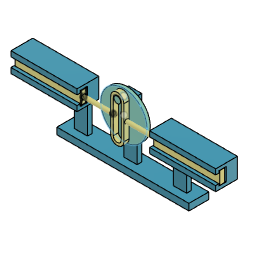
Scotch Yoke Mechanism v9 (Autodesk Fusion 360 design; units mm, degrees)
Autodesk Fusion 360 part; units mm, degrees
sketch "holder base" plane through (0, 0, 0) normal (0, 0, 1) x (1, 0, 0) in component "Holder"
  line L0 (-100, -15) -> (100, -15)
  line L1 (100, -15) -> (100, 15)
  line L2 (100, 15) -> (-100, 15)
  line L3 (-100, 15) -> (-100, -15)
  line L4 (-100, -15) -> (100, 15) construction
  line L5 (100, -15) -> (-100, 15) construction
  constraint horizontal L0
  constraint perpendicular L0 L1
  constraint parallel L0 L2
  constraint parallel L1 L3
  constraint coincident L4 origin
  constraint coincident L5 origin
extrude "Extrude1" add sketch "holder base" along normal blind 10 makes body 1 in component "Holder"
sketch "crank holder base" plane through (0, 0, 10) normal (0, 0, 1) x (-1, 0, 0) in component "Holder"
  line L0 (100, -15) -> (100, 15)
  line L1 (100, 15) -> (-100, 15)
  line L2 (-100, 15) -> (-100, -15)
  line L3 (-100, -15) -> (100, -15)
  line L4 (-10, 3.5) -> (10, 3.5)
  line L5 (10, 3.5) -> (10, -3.5)
  line L6 (10, -3.5) -> (-10, -3.5)
  line L7 (-10, -3.5) -> (-10, 3.5)
  line L8 (-10, 3.5) -> (10, -3.5) construction
  line L9 (10, 3.5) -> (-10, -3.5) construction
  dimension "d3" = 20
  dimension "d4" = 7
  constraint horizontal L4
  constraint perpendicular L4 L5
  constraint parallel L4 L6
  constraint parallel L5 L7
  constraint coincident L8 origin
  constraint coincident L9 origin
  measures "d3" distance of L5.end L6.end
  measures "d4" distance of L4.end L5.end
extrude "Extrude2" add sketch "crank holder base" along normal blind 150 contours L4 L5 L6 L7 bodies 1 in component "Holder"
sketch "slider holder base" plane through (0, 0, 10) normal (0, 0, 1) x (-1, 0, 0) in component "Holder"
  line L0 (-10, -3.5) -> (-10, 3.5)
  line L1 (-10, 3.5) -> (10, 3.5)
  line L2 (10, 3.5) -> (10, -3.5)
  line L3 (10, -3.5) -> (-10, -3.5)
  line L4 (100, -15) -> (100, 15)
  line L5 (100, 15) -> (-100, 15)
  line L6 (-100, 15) -> (-100, -15)
  line L7 (-100, -15) -> (100, -15)
  line L8 (-85, 3.5) -> (-65, 3.5)
  line L9 (-65, 3.5) -> (-65, -3.5)
  line L10 (-65, -3.5) -> (-85, -3.5)
  line L11 (-85, -3.5) -> (-85, 3.5)
  line L12 (-85, 3.5) -> (-65, -3.5) construction
  line L13 (-65, 3.5) -> (-85, -3.5) construction
  line L14 (0, -15) -> (0, 15)
  line L15 (65, -3.5) -> (85, -3.5)
  line L16 (85, 3.5) -> (65, 3.5)
  line L17 (85, -3.5) -> (85, 3.5)
  line L18 (65, 3.5) -> (65, -3.5)
  point P0 (-75, 0)
  dimension "d7" = 20
  dimension "d8" = 7
  constraint horizontal L8
  constraint perpendicular L8 L9
  constraint parallel L8 L10
  constraint parallel L9 L11
  constraint coincident L12 P0
  constraint coincident L13 P0
  constraint midpoint L7 L14.start
  constraint midpoint L5 L14.end
  constraint symmetric L8.start L14 L16.start
  constraint symmetric L8.end L14 L16.end
  constraint symmetric L9.end L14 L15.start
  constraint symmetric L10.end L14 L15.end
  measures "d7" distance of L9.end L10.end
  measures "d8" distance of L8.end L9.end
extrude "Extrude3" add sketch "slider holder base" along normal blind 110 contours L8 L9 L10 L11 | L15 L16 L17 L18 bodies 1 in component "Holder"
sketch "crank holder" plane through (0, -3.5, 0) normal (0, -1, 0) x (1, 0, 0) in component "Holder"
  line L0 (-10, 10) -> (10, 10)
  line L1 (10, 10) -> (10, 160)
  line L2 (10, 160) -> (-10, 160)
  line L3 (-10, 160) -> (-10, 10)
  circle A0 centre (0, 135) radius 5
  dimension "d11" = 10
  measures "d11" diameter of A0
extrude "Extrude4" add sketch "crank holder" along normal blind 10 contours A0 bodies 1 in component "Holder"
sketch "crank" plane through (0, -13.5, 0) normal (0, -1, 0) x (1, 0, 0) in component "Crank"
  circle A0 centre (0, 135) radius 5
  circle A1 centre (0, 135) radius 35
  circle A2 centre (0, 160) radius 5
  dimension "d14" = 10
  constraint concentric A0 A1
  measures "d14" diameter of A2
extrude "Extrude1'" add sketch "crank" against normal blind 5 separate body contours A1 | A2 makes body 2 in component "Crank"
move_face "OffsetFaces1" offset -0.3 1 faces at (-4.6985, -10.1667, 133.2899) on bodies 1 in component "Holder"
extrude "Extrude2'" add sketch "crank" along normal blind 10 contours A2 bodies 2 in component "Crank"
sketch "slider holder side" plane through (0, -3.5, 0) normal (0, -1, 0) x (1, 0, 0) in component "Holder"
  line L0 (-85, 10) -> (-65, 10)
  line L1 (-65, 10) -> (-65, 120)
  line L2 (-65, 120) -> (-85, 120)
  line L3 (-85, 120) -> (-85, 10)
  line L4 (-55, 120) -> (-155, 120)
  line L5 (-155, 120) -> (-155, 150)
  line L6 (-155, 150) -> (-55, 150)
  line L7 (-55, 150) -> (-55, 120)
  line L8 (0, 160) -> (0, 10)
  line L9 (155, 150) -> (55, 150)
  line L10 (55, 150) -> (55, 120)
  line L11 (55, 120) -> (155, 120)
  line L12 (155, 120) -> (155, 150)
  line L13 (-155, 150) -> (-55, 150)
  line L14 (-55, 150) -> (-55, 145)
  line L15 (-55, 145) -> (-155, 145)
  line L16 (-155, 145) -> (-155, 150)
  line L17 (-55, 120) -> (-155, 120)
  line L18 (-155, 120) -> (-155, 125)
  line L19 (-155, 125) -> (-55, 125)
  line L20 (-55, 125) -> (-55, 120)
  line L21 (55, 145) -> (155, 145)
  line L22 (155, 125) -> (55, 125)
  dimension "d20" = 100
  dimension "d21" = 30
  dimension "d24" = 5
  dimension "d25" = 5
  constraint horizontal L4
  constraint vertical L5
  constraint horizontal L6
  constraint vertical L7
  constraint vertical L8
  constraint symmetric L4.start L8 L10.end
  constraint symmetric L4.end L8 L11.end
  constraint symmetric L5.end L8 L9.start
  constraint symmetric L6.end L8 L9.end
  constraint horizontal L13
  constraint vertical L14
  constraint horizontal L15
  constraint vertical L16
  constraint coincident L7 L14.end
  constraint horizontal L17
  constraint vertical L18
  constraint horizontal L19
  constraint vertical L20
  constraint symmetric L8 L14.end L21.start
  constraint symmetric L8 L15.end L21.end
  constraint symmetric L8 L18.end L22.start
  constraint symmetric L8 L19.end L22.end
  measures "d20" distance of L4.start L4.end
  measures "d21" distance of L4.start L6.end
  measures "d24" distance of L5.end L15.end
  measures "d25" distance of L4.start L19.end
extrude "Extrude5" add sketch "slider holder side" against normal blind 7 contours L2 L4 L5 L7 L17 L18 L19 L20 | L5 L7 L15 L19 | L5 L6 L7 L13 L14 L15 L16 | L9 L10 L12 L21 | L10 L12 L21 L22 | L10 L11 L12 L22 bodies 1 in component "Holder"
extrude "Extrude6" add sketch "slider holder side" along normal blind 20 contours L2 L4 L5 L7 L17 L18 L19 L20 | L5 L6 L7 L13 L14 L15 L16 | L9 L10 L12 L21 | L10 L11 L12 L22 bodies 1 in component "Holder"
sketch "slider center" plane through (0, -23.5, 0) normal (0, -1, 0) x (1, 0, 0) in component "Slider"
  circle A0 centre (0, 160) radius 5
  line L0 (0, 170) -> (0, 100)
  line L1 (-10, 160) -> (-10, 110)
  line L2 (0, 100) -> (0, 170) construction
  line L3 (10, 160) -> (10, 110)
  line L4 (-10, 135) -> (10, 135) construction
  arc A1 (-6, 110) -> (6, 110) centre (0, 110) ccw
  line L5 (6, 160) -> (6, 110)
  arc A2 (6, 160) -> (-6, 160) centre (0, 160) ccw
  line L6 (-6, 110) -> (-6, 160)
  arc A3 (-10, 110) -> (10, 110) centre (0, 110) ccw
  line L7 (10, 160) -> (10, 110)
  arc A4 (10, 160) -> (-10, 160) centre (0, 160) ccw
  line L8 (-10, 110) -> (-10, 160)
  dimension "d29" = 70
  constraint vertical L0
  constraint vertical L1
  constraint vertical L2
  constraint coincident L1 L4.start
  constraint coincident L3 L4.end
  constraint tangent A1 L6
  constraint tangent A1 L5
  constraint tangent L5 A2
  constraint tangent A2 L6
  constraint tangent L7 A4
  constraint tangent A3 L8
  constraint tangent A3 L7
  constraint tangent A4 L8
  measures "d29" distance of L0.start L0.end
extrude "Extrude1''" add sketch "slider center" against normal blind 8 separate body contours L0 L1 A1 A2 L6 A3 A4 L8 | L0 L3 A1 L5 A2 A3 L7 A4 makes body 3
sketch "Sketch2" plane through (10, 0, 0) normal (1, 0, 0) x (0, 1, 0) in component "Slider"
  line L0 (-23.5, 160) -> (-23.5, 110)
  line L1 (-23.5, 110) -> (-15.5, 110)
  line L2 (-15.5, 110) -> (-15.5, 160)
  line L3 (-15.5, 160) -> (-23.5, 160)
copy_body "CutPasteBodies1" bodies 3 removing the originals makes body 4 in component "Slider"
sketch "slider right link" plane through (10, 0, 0) normal (1, 0, 0) x (0, 1, 0) in component "Slider"
  line L0 (-19.5, 160) -> (-19.5, 110) construction
  circle A0 centre (-19.5, 135) radius 3
  dimension "d34" = 6
  constraint vertical L0
  constraint midpoint L0 A0.centre
  measures "d34" diameter of A0
extrude "Extrude1'''" add sketch "slider right link" along normal blind 45 bodies 4 in component "Slider"
sketch "slider left link" plane through (-10, 0, 0) normal (-1, 0, 0) x (0, -1, 0) in component "Slider"
  line L0 (23.5, 110) -> (23.5, 160)
  line L1 (23.5, 160) -> (15.5, 160)
  line L2 (15.5, 160) -> (15.5, 110)
  line L3 (15.5, 110) -> (23.5, 110)
  line L4 (19.5, 160) -> (19.5, 110) construction
  circle A0 centre (19.5, 135) radius 3
  dimension "d37" = 6
  constraint midpoint L1 L4.start
  constraint midpoint L3 L4.end
  constraint midpoint L4 A0.centre
  measures "d37" diameter of A0
extrude "Extrude2''" add sketch "slider left link" along normal blind 45 contours A0 bodies 4 in component "Slider"
sketch "slider left" plane through (-55, 0, 0) normal (-1, 0, 0) x (0, -1, 0) in component "Slider"
  circle A0 centre (19.5, 135) radius 3
  line L0 (23.5, 125) -> (15.5, 125)
  line L1 (15.5, 125) -> (15.5, 145)
  line L2 (15.5, 145) -> (23.5, 145)
  line L3 (23.5, 145) -> (23.5, 125)
  line L4 (23.5, 125) -> (15.5, 145) construction
  line L5 (15.5, 125) -> (23.5, 145) construction
  point P0 (19.5, 135)
  dimension "d40" = 8
  dimension "d41" = 20
  constraint horizontal L0
  constraint perpendicular L0 L1
  constraint parallel L0 L2
  constraint parallel L1 L3
  constraint coincident L4 P0
  constraint coincident L5 P0
  constraint coincident P0 A0.centre
  measures "d40" distance of L1.end L2.end
  measures "d41" distance of L0.end L1.end
extrude "Extrude4'" add sketch "slider left" along normal blind 100 contours A0 | L0 L1 L2 L3 bodies 4 in component "Slider"
sketch "slider right" plane through (55, 0, 0) normal (1, 0, 0) x (0, 1, 0) in component "Slider"
  circle A0 centre (-19.5, 135) radius 3
  line L0 (-15.5, 125) -> (-23.5, 125)
  line L1 (-23.5, 125) -> (-23.5, 145)
  line L2 (-23.5, 145) -> (-15.5, 145)
  line L3 (-15.5, 145) -> (-15.5, 125)
  line L4 (-15.5, 125) -> (-23.5, 145) construction
  line L5 (-23.5, 125) -> (-15.5, 145) construction
  point P0 (-19.5, 135)
  dimension "d46" = 8
  dimension "d47" = 20
  constraint horizontal L0
  constraint perpendicular L0 L1
  constraint parallel L0 L2
  constraint parallel L1 L3
  constraint coincident L4 P0
  constraint coincident L5 P0
  constraint coincident P0 A0.centre
  measures "d46" distance of L1.end L2.end
  measures "d47" distance of L0.end L1.end
extrude "Extrude5'" add sketch "slider right" along normal blind 100 contours A0 | L0 L1 L2 L3 bodies 4 in component "Slider"
move_face "OffsetFaces1'" offset -0.3 4 faces at (88.3333, -23.5, 131.6667) (88.3333, -20.8333, 145) (88.3333, -15.5, 138.3333) (88.3333, -18.1667, 125) on bodies 4 in component "Slider"
move_face "OffsetFaces2" offset -0.3 4 faces at (-88.3333, -23.5, 138.3333) (-121.6667, -20.8333, 145) (-88.3333, -20.8333, 125) (-88.3333, -15.5, 131.6667) on bodies 4 in component "Slider"
extrude "Extrude7" add 1 faces at (-121.6667, -3.5, 131.6667) along direction (0, -1, 0) blind 10 on bodies 1 bodies 1 in component "Holder"
extrude "Extrude8" add 1 faces at (121.6667, -3.5, 131.6667) along direction (0, -1, 0) blind 10 on bodies 1 bodies 1 in component "Holder"
extrude "Extrude9" add 4 faces at (-121.6667, -23.5, 148.3333) (-121.6667, -23.5, 123.3333) (88.3333, -23.5, 148.3333) (88.3333, -23.5, 123.3333) along direction (0, -1, 0) blind 6 on bodies 1 bodies 1 in component "Holder"
sketch "slider rail right bottom" plane through (0, 0, 125) normal (0, 0, 1) x (-1, 0, 0) in component "Holder"
  line L0 (-155, 13.5) -> (-55, 13.5)
  line L1 (-55, 13.5) -> (-55, 29.5)
  line L2 (-55, 29.5) -> (-155, 29.5)
  line L3 (-155, 29.5) -> (-155, 13.5)
  line L4 (-155, 29.5) -> (-55, 29.5)
  line L5 (-55, 29.5) -> (-55, 24.5)
  line L6 (-55, 24.5) -> (-155, 24.5)
  line L7 (-155, 24.5) -> (-155, 29.5)
  dimension "d58" = 100
  dimension "d59" = 5
  constraint horizontal L4
  constraint vertical L5
  constraint horizontal L6
  constraint vertical L7
  constraint coincident L2.end L3.start
  measures "d58" distance of L2.end L1.end
  measures "d59" distance of L2.end L6.end
sketch "slider rail right top" plane through (0, 0, 145) normal (0, 0, -1) x (1, 0, 0) in component "Holder"
  line L0 (55, 13.5) -> (155, 13.5)
  line L1 (155, 13.5) -> (155, 29.5)
  line L2 (155, 29.5) -> (55, 29.5)
  line L3 (55, 29.5) -> (55, 13.5)
  line L4 (155, 29.5) -> (55, 29.5)
  line L5 (55, 29.5) -> (55, 24.5)
  line L6 (55, 24.5) -> (155, 24.5)
  line L7 (155, 24.5) -> (155, 29.5)
  dimension "d60" = 100
  dimension "d61" = 5
  constraint horizontal L4
  constraint vertical L5
  constraint horizontal L6
  constraint vertical L7
  constraint coincident L1.end L2.start
  measures "d60" distance of L1.end L2.end
  measures "d61" distance of L1.end L6.end
extrude "Extrude10" add sketch "slider rail right bottom" along normal blind 3 contours L1 L2 L3 L4 L5 L6 L7 bodies 1 in component "Holder"
extrude "Extrude11" add sketch "slider rail right top" along normal blind 3 contours L1 L2 L3 L4 L5 L6 L7 bodies 1 in component "Holder"
sketch "slider rail left bottom" plane through (0, 0, 125) normal (0, 0, 1) x (-1, 0, 0) in component "Holder"
  line L0 (55, 13.5) -> (155, 13.5)
  line L1 (155, 13.5) -> (155, 29.5)
  line L2 (155, 29.5) -> (55, 29.5)
  line L3 (55, 29.5) -> (55, 13.5)
  line L4 (155, 29.5) -> (55, 29.5)
  line L5 (55, 29.5) -> (55, 24.5)
  line L6 (55, 24.5) -> (155, 24.5)
  line L7 (155, 24.5) -> (155, 29.5)
  dimension "d66" = 100
  dimension "d67" = 5
  constraint horizontal L4
  constraint vertical L5
  constraint horizontal L6
  constraint vertical L7
  constraint coincident L1.end L2.start
  measures "d66" distance of L1.end L2.end
  measures "d67" distance of L1.end L6.end
sketch "slider rail left top" plane through (0, 0, 145) normal (0, 0, -1) x (1, 0, 0) in component "Holder"
  line L0 (-155, 13.5) -> (-55, 13.5)
  line L1 (-55, 13.5) -> (-55, 29.5)
  line L2 (-55, 29.5) -> (-155, 29.5)
  line L3 (-155, 29.5) -> (-155, 13.5)
  line L4 (-155, 29.5) -> (-55, 29.5)
  line L5 (-55, 29.5) -> (-55, 24.5)
  line L6 (-55, 24.5) -> (-155, 24.5)
  line L7 (-155, 24.5) -> (-155, 29.5)
  dimension "d68" = 100
  dimension "d69" = 5
  constraint horizontal L4
  constraint vertical L5
  constraint horizontal L6
  constraint vertical L7
  constraint coincident L2.end L3.start
  measures "d68" distance of L2.end L1.end
  measures "d69" distance of L2.end L6.end
extrude "Extrude12" add sketch "slider rail left bottom" along normal blind 3 contours L1 L2 L3 L4 L5 L6 L7 bodies 1 in component "Holder"
extrude "Extrude13" add sketch "slider rail left top" along normal blind 3 contours L1 L2 L3 L4 L5 L6 L7 bodies 1 in component "Holder"
extrude "Extrude14" add sketch "crank holder base" along normal blind 60 bodies 1 in component "Holder"
extrude "Extrude15" cut sketch "holder base" along normal blind 60 bodies 1 in component "Holder"
component "Holder" placed x (1, 0, 0) y (0, 1, 0) z (0, 0, 1) at (0, 0, -60)
component "Crank" placed x (1, 0, 0) y (0, 1, 0) z (0, 0, 1) at (0, 0, -60)
component "Slider" placed x (1, 0, 0) y (0, 1, 0) z (0, 0, 1) at (0, 0, -60)
named bodies: "holder", "crank", "slider"
